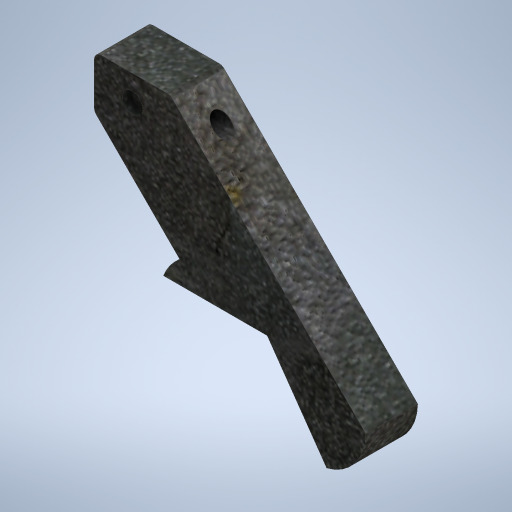
# Autodesk Inventor part: Ramię ze szczękami
Saved by Autodesk Inventor 2024 (Build 280153000, 153)
## iProperties
Created: 2024-04-14
Part Number: Ramię ze szczękami
Material: Steel
Document SubType Name: Modeling
Designer: HP
Density: 7.85 g/cm^3
Appearance: Plate
Author: HP
Autodesk Inventor part; units mm, degrees
ref_plane "YZ Plane" through (0, 0, 0) normal (1, 0, 0) x (0, 1, 0)
ref_plane "XZ Plane" through (0, 0, 0) normal (0, 1, 0) x (-1, 0, 0)
ref_plane "XY Plane" through (0, 0, 0) normal (0, 0, 1) x (1, 0, 0)
sketch "Sketch1" plane through (0, 0, 0) normal (0, 0, 1) x (1, 0, 0)
  line L0 (0, 0) -> (0, 15)
  line L1 (0, 15) -> (22, 15)
  line L2 (22, 15) -> (78.5685, -41.5685)
  line L3 (0, 0) -> (24.7487, -24.7487)
  line L4 (0, 0) -> (35, 0) construction
  line L5 (0, 15) -> (0, 7.5) construction
  line L6 (11.1378, 7.6884) -> (50.0287, -31.2025) construction
  line L7 (11.1378, 7.6884) -> (66.1378, 7.6884) construction
  line L8 (50.0287, -31.2025) -> (67.2359, -55.777)
  line L9 (50.0287, -31.2025) -> (80.0287, -31.2025) construction
  line L10 (50.0287, -31.2025) -> (20.0287, -31.2025)
  arc A0 (24.7487, -24.7487) -> (20.0287, -31.2025) centre (34.0582, -36.5103) ccw
  arc A1 (67.2359, -55.777) -> (78.5685, -41.5685) centre (63.5723, -41.2313) ccw
  dimension "d0" = 15
  dimension "d1" = 22
  dimension "d2" = 80
  dimension "d3" = 135
  dimension "d4" = 35
  dimension "d5" = 45
  dimension "d6" = 55
  dimension "d7" = 45
  dimension "d8" = 30
  dimension "d9" = 55
  dimension "d10" = 30
  dimension "d11" = 15
  dimension "d12" = 15
  constraints: 22 end point, 4 horizontal, 4 point on circle, 3 equal length, 2 centre point, 1 midpoint, 1 perpendicular, 1 vertical
  measures "d0" distance of L0.start L0.end
  measures "d1" distance of L0.end L1.end
  measures "d2" distance of L1.end L2.end
  measures "d3" angle of L1 L2
  measures "d4" distance of L0.start L3.end
  measures "d5" angle of L3 L4
  measures "d6" distance of L6.start L6.end
  measures "d7" angle of L6 L7
  measures "d8" distance of L6.end L8.end
  measures "d9" angle of L8 L9
  measures "d10" distance of L6.end L10.end
  measures "d11" radius of A0
  measures "d12" radius of A1
extrude "Extrusion1" add sketch "Sketch1" along normal blind 15
sketch "Sketch2" plane through (0, 0, 0) normal (-1, 0, 0) x (0, 0, 1)
  line L0 (0, -41.5685) -> (0, 15) construction
  line L1 (0, 15) -> (7.5, 15) construction
  line L2 (0, 15) -> (15, 15) construction
  line L3 (7.5, 15) -> (7.5, 7.5) construction
  circle A0 centre (7.5, 7.5) radius 2.5
  point P0 (0, 0)
  dimension "d15" = 7.5
  dimension "d16" = 7.5
  dimension "d17" = 5
  constraints: 4 end point, 1 centre point, 1 coincident, 1 midpoint, 1 vertical
  measures "d15" distance of L0.end L1.end
  measures "d16" distance of L1.end L3.end
  measures "d17" diameter of A0
extrude "Extrusion2" cut sketch "Sketch2" against normal blind 33
fillet "Fillet1" radius 2 2 edges at (0, 15, 7.5) (0, 0, 7.5)
fillet "Fillet2" radius 2 1 edges at (22, 15, 7.5)
sketch "Sketch3" plane through (0, 0, 15) normal (0, 0, 1) x (1, 0, 0)
  line L0 (21.1716, 15) -> (2, 15) construction
  line L1 (6.35, 15) -> (6.35, 7.5) construction
  line L2 (0, 13) -> (0, 0.8284) construction
  line L3 (0, 7.5) -> (11, 7.5) construction
  line L4 (0, 7.5) -> (11, 7.5) construction
  circle A0 centre (11, 7.5) radius 3
  point P0 (0, 0)
  dimension "d22" = 7.5
  dimension "d23" = 11
  dimension "d24" = 0
  dimension "d25" = 6
  constraints: 6 end point, 2 point on line, 1 centre point, 1 coincident, 1 collinear, 1 horizontal, 1 perpendicular, 1 vertical
  measures "d22" distance of L1.start L1.end
  measures "d23" distance of L3.start L3.end
  measures "d24" distance between parallel lines of L3 L4
  measures "d25" diameter of A0
extrude "Extrusion3" cut sketch "Sketch3" against normal blind 3
sketch "Sketch4" plane through (0, 0, 0) normal (0, 0, -1) x (-1, 0, 0)
  line L0 (-21.1716, 15) -> (-2, 15) construction
  line L1 (-4.7625, 15) -> (-4.7625, 7.5) construction
  line L2 (-4.7625, 15) -> (2.7375, 15) construction
  line L3 (0, 13) -> (0, 0.8284) construction
  line L4 (0, 7.5) -> (-11, 7.5) construction
  line L5 (0, 7.5) -> (11, 7.5) construction
  circle A0 centre (-11, 7.5) radius 3
  point P0 (0, 0)
  dimension "d28" = 7.5
  dimension "d29" = 90
  dimension "d30" = 11
  dimension "d31" = 180
  dimension "d32" = 6
  constraints: 8 end point, 2 equal length, 2 horizontal, 2 perpendicular, 2 point on line, 1 centre point, 1 coincident
  measures "d28" distance of L1.start L1.end
  measures "d29" angle of L1 L2
  measures "d30" distance of L4.start L4.end
  measures "d31" angle of L4 L5
  measures "d32" diameter of A0
extrude "Extrusion4" cut sketch "Sketch4" against normal blind 3
body "Solid1"
